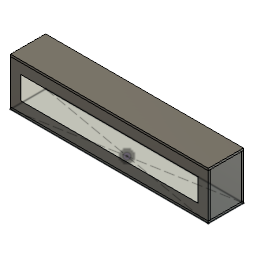
initial_3d_design (Autodesk Fusion 360 design; units mm, degrees)
part number: 2026-03-02-16-33-59-014
part number: 2026-03-03-11-30-51-863
part number: 2026-03-03-11-31-05-266
part number: 2026-03-03-11-31-17-109
part number: 2026-03-03-11-31-19-151
part number: 2026-03-03-11-31-20-913
part number: 2026-03-03-11-31-23-209
part number: 2026-03-03-11-31-25-857
part number: 2026-03-03-11-31-27-912
part number: 2026-03-03-11-31-30-099
Autodesk Fusion 360 part; units mm, degrees
sketch "Base/Top" plane through (0, 0, 0) normal (0, 1, 0) x (1, 0, 0)
  line L0 (143, 25.5) -> (-143, 25.5)
  line L1 (-143, 25.5) -> (-143, -25.5)
  line L2 (-143, -25.5) -> (143, -25.5)
  line L3 (143, -25.5) -> (143, 25.5)
  line L4 (143, 25.5) -> (-143, -25.5) construction
  line L5 (-143, 25.5) -> (143, -25.5) construction
  dimension "d12" = 286
  dimension "d13" = 51
  constraint horizontal L0
  constraint perpendicular L0 L1
  constraint parallel L0 L2
  constraint parallel L1 L3
  constraint coincident L4 origin
  constraint coincident L5 origin
  measures "d12" distance of L1.end L2.end
  measures "d13" distance of L0.end L1.end
sketch "Front" plane through (0, 0, 0) normal (0, 0, 1) x (1, 0, 0)
  line L0 (128, 16.5) -> (-128, 16.5)
  line L1 (-128, 16.5) -> (-128, -16.5)
  line L2 (-128, -16.5) -> (128, -16.5)
  line L3 (128, -16.5) -> (128, 16.5)
  line L4 (128, 16.5) -> (-128, -16.5) construction
  line L5 (-128, 16.5) -> (128, -16.5) construction
  line L6 (143, 31.5) -> (-143, 31.5)
  line L7 (-143, 31.5) -> (-143, -31.5)
  line L8 (-143, -31.5) -> (143, -31.5)
  line L9 (143, -31.5) -> (143, 31.5)
  line L10 (143, 31.5) -> (-143, -31.5) construction
  line L11 (-143, 31.5) -> (143, -31.5) construction
  dimension "d15" = 256
  dimension "d16" = 33
  dimension "d17" = 286
  dimension "d18" = 63
  constraint horizontal L0
  constraint perpendicular L0 L1
  constraint parallel L0 L2
  constraint parallel L1 L3
  constraint coincident L4 origin
  constraint coincident L5 origin
  constraint horizontal L6
  constraint perpendicular L6 L7
  constraint parallel L6 L8
  constraint parallel L7 L9
  constraint coincident L10 origin
  constraint coincident L11 origin
  measures "d15" distance of L1.end L2.end
  measures "d16" distance of L0.end L1.end
  measures "d17" distance of L7.end L8.end
  measures "d18" distance of L6.end L7.end
sketch "Lights" plane through (0, 0, 0) normal (0, 0, 1) x (1, 0, 0)
  line L0 (128, 16.5) -> (-128, 16.5)
  line L1 (-128, 16.5) -> (-128, -16.5)
  line L2 (-128, -16.5) -> (128, -16.5)
  line L3 (128, -16.5) -> (128, 16.5)
  line L4 (128, 16.5) -> (-128, -16.5) construction
  line L5 (-128, 16.5) -> (128, -16.5) construction
  line L6 (0, 0) -> (128, 0) construction
  line L7 (0, 0) -> (0, 16.5) construction
  dimension "d19" = 256
  dimension "d20" = 33
  constraint horizontal L0
  constraint perpendicular L0 L1
  constraint parallel L0 L2
  constraint parallel L1 L3
  constraint coincident L4 L6.start
  constraint coincident L5 L6.start
  constraint coincident L6.start L7.start
  constraint midpoint L3 L6.end
  constraint midpoint L0 L7.end
  measures "d19" distance of L1.end L2.end
  measures "d20" distance of L0.end L1.end
sketch "Back" plane through (0, 0, 0) normal (0, 0, 1) x (1, 0, 0)
  line L0 (143, 31.5) -> (-143, 31.5)
  line L1 (-143, 31.5) -> (-143, -31.5)
  line L2 (-143, -31.5) -> (143, -31.5)
  line L3 (143, -31.5) -> (143, 31.5)
  line L4 (143, 31.5) -> (-143, -31.5) construction
  line L5 (-143, 31.5) -> (143, -31.5) construction
  line L6 (143, -31.5) -> (128, -31.5) construction
  line L7 (128, -31.5) -> (128, -24) construction
  line L8 (128, -24) -> (118, -24)
  line L9 (118, -24) -> (118, -21.5)
  line L10 (118, -21.5) -> (128, -21.5)
  line L11 (128, -21.5) -> (128, -24)
  line L12 (118, -24) -> (110.5, -24) construction
  line L13 (110.5, -24) -> (98.5, -24)
  line L14 (98.5, -24) -> (98.5, -12)
  line L15 (98.5, -12) -> (110.5, -12)
  line L16 (110.5, -12) -> (110.5, -24)
  line L17 (128, -21.5) -> (123, -21.5) construction
  line L18 (123, -21.5) -> (123, -16.5) construction
  circle A0 centre (123, -16.5) radius 2.5
  dimension "d21" = 286
  dimension "d22" = 63
  dimension "d23" = 15
  dimension "d24" = 7.5
  dimension "d27" = 10
  dimension "d28" = 2.5
  dimension "d29" = 7.5
  dimension "d30" = 12
  dimension "d31" = 12
  dimension "d32" = 5
  dimension "d34" = 5
  constraint horizontal L0
  constraint perpendicular L0 L1
  constraint parallel L0 L2
  constraint parallel L1 L3
  constraint coincident L4 origin
  constraint coincident L5 origin
  constraint perpendicular L3 L6
  constraint perpendicular L2 L7
  constraint horizontal L8
  constraint vertical L9
  constraint horizontal L10
  constraint vertical L11
  constraint perpendicular L9 L12
  constraint horizontal L13
  constraint vertical L14
  constraint horizontal L15
  constraint vertical L16
  constraint midpoint L10 L17.end
  constraint perpendicular L17 L18
  constraint coincident L18.end A0.centre
  measures "d21" distance of L1.end L2.end
  measures "d22" distance of L0.end L1.end
  measures "d23" distance of L2.end L6.end
  measures "d24" distance of L6.end L7.end
  measures "d27" distance of L7.end L8.end
  measures "d28" distance of L7.end L10.end
  measures "d29" distance of L8.end L12.end
  measures "d30" distance of L12.end L13.end
  measures "d31" distance of L12.end L15.end
  measures "d32" distance of L17.end L18.end
  measures "d34" diameter of A0
sketch "Sides" plane through (0, 0, 0) normal (1, 0, 0) x (0, 0, -1)
  line L0 (22.5, 31.5) -> (-22.5, 31.5)
  line L1 (-22.5, 31.5) -> (-22.5, -31.5)
  line L2 (-22.5, -31.5) -> (22.5, -31.5)
  line L3 (22.5, -31.5) -> (22.5, 31.5)
  line L4 (22.5, 31.5) -> (-22.5, -31.5) construction
  line L5 (-22.5, 31.5) -> (22.5, -31.5) construction
  dimension "d35" = 45
  dimension "d36" = 63
  constraint horizontal L0
  constraint perpendicular L0 L1
  constraint parallel L0 L2
  constraint parallel L1 L3
  constraint coincident L4 origin
  constraint coincident L5 origin
  measures "d35" distance of L1.end L2.end
  measures "d36" distance of L0.end L1.end
sketch "Esp32" plane through (0, 0, 0) normal (0, 1, 0) x (1, 0, 0)
  line L0 (-28.5, -14.25) -> (28.5, -14.25)
  line L1 (28.5, -14.25) -> (28.5, 14.25)
  line L2 (28.5, 14.25) -> (-28.5, 14.25)
  line L3 (-28.5, 14.25) -> (-28.5, -14.25)
  line L4 (-28.5, -14.25) -> (28.5, 14.25) construction
  line L5 (28.5, -14.25) -> (-28.5, 14.25) construction
  dimension "d37" = 57
  dimension "d38" = 28.5
  constraint horizontal L0
  constraint perpendicular L0 L1
  constraint parallel L0 L2
  constraint parallel L1 L3
  constraint coincident L4 origin
  constraint coincident L5 origin
  measures "d37" distance of L1.end L2.end
  measures "d38" distance of L0.end L1.end
sketch "Button" plane through (0, 0, 0) normal (0, 0, 1) x (1, 0, 0)
  line L0 (-6, 6) -> (6, 6)
  line L1 (6, 6) -> (6, -6)
  line L2 (6, -6) -> (-6, -6)
  line L3 (-6, -6) -> (-6, 6)
  line L4 (-6, 6) -> (6, -6) construction
  line L5 (6, 6) -> (-6, -6) construction
  circle A0 centre (0, 0) radius 2.6
  dimension "d39" = 12
  dimension "d40" = 12
  dimension "d41" = 5.2
  constraint horizontal L0
  constraint perpendicular L0 L1
  constraint parallel L0 L2
  constraint parallel L1 L3
  constraint coincident L4 A0.centre
  constraint coincident L5 A0.centre
  constraint coincident A0.centre origin
  measures "d39" distance of L1.end L2.end
  measures "d40" distance of L0.end L1.end
  measures "d41" diameter of A0
extrude "Extrude1" add sketch "Base/Top" along normal blind 3 makes body 1
copy_body "CopyPasteBodies1" bodies 1 makes body 2
extrude "Extrude2" add sketch "Front" along normal blind 3 separate body makes body 3
extrude "Extrude3" add sketch "Lights" along normal blind 15 separate body makes body 4
extrude "Extrude4" add sketch "Back" along normal blind 3 separate body makes body 5
extrude "Extrude5" add sketch "Sides" along normal blind 3 separate body makes body 6
copy_body "CopyPasteBodies2" bodies 6 makes body 7
extrude "Extrude6" add sketch "Esp32" along normal blind 3 separate body makes body 8
extrude "Extrude7" add sketch "Button" along normal blind 6.5 separate body makes body 9
extrude "Extrude8" add sketch "Button" along normal blind 8.5 separate body contours A0 makes body 10
combine "Combine1" operation add target body 9 tool bodies 10
copy_body "Body->Comp1" bodies 1 removing the originals makes body 11 in component "Base"
copy_body "Body->Comp2" bodies 3 removing the originals makes body 12 in component "Front"
copy_body "Body->Comp3" bodies 2 removing the originals makes body 13 in component "Top"
copy_body "Body->Comp4" bodies 4 removing the originals makes body 14 in component "Lights"
copy_body "Body->Comp5" bodies 5 removing the originals makes body 15 in component "Back"
copy_body "Body->Comp6" bodies 6 removing the originals makes body 16 in component "LeftSide"
copy_body "Body->Comp7" bodies 7 removing the originals makes body 17 in component "RightSide"
copy_body "Body->Comp8" bodies 8 removing the originals makes body 18 in component "ESP32"
copy_body "Body->Comp9" bodies 9 removing the originals makes body 19 in component "Button"
fillet "Fillet1" radius 1 4 edges at (118, -21.5, 1.5) (118, -24, 1.5) (128, -24, 1.5) (128, -21.5, 1.5) on bodies 15 in component "Back"
fillet "Fillet1'" radius 1 4 edges at (0, -6, 6.5) (6, 0, 6.5) (-6, 0, 6.5) (0, 6, 6.5) on bodies 19 in component "Button"
move_body "Move1" bodies 18 to x (1, 0, 0) y (0, 1, 0) z (0, 0, 1) at (0, 100, 0) in component "ESP32"
move_body "Move1'" bodies 13 to x (1, 0, 0) y (0, 1, 0) z (0, 0, 1) at (0, 90, 0) in component "Top"
component "Base" placed x (1, 0, 0) y (0, 1, 0) z (0, 0, 1) at (0, 0, 0)
component "Front" placed x (1, 0, 0) y (0, 1, 0) z (0, 0, 1) at (0, 34.5, 22.5)
component "Top" placed x (1, 0, 0) y (0, 1, 0) z (0, 0, 1) at (0, -24, 0)
component "Lights" placed x (1, 0, 0) y (0, 1, 0) z (0, 0, 1) at (0, 34.5, 10.5)
component "Back" placed x (-1, 0, 0) y (0, 1, 0) z (0, 0, -1) at (0, 34.5, -22.5)
component "LeftSide" placed x (1, 0, 0) y (0, 1, 0) z (0, 0, 1) at (-143, 34.5, 0)
component "RightSide" placed x (1, 0, 0) y (0, 1, 0) z (0, 0, 1) at (140, 34.5, 0)
component "ESP32" placed x (1, 0, 0) y (0, 1, 0) z (0, 0, 1) at (-111.5, -97, -4.25)
component "Button" placed x (-1, 0, 0) y (0, 1, 0) z (0, 0, -1) at (-104.5, 16.5, -20)
equation "lights_length = 256 mm"
equation "lights_width = 33 mm"
equation "lights_depth = 15 mm"
equation "housing_buffer = 15 mm"
equation "mat_thickness = 3 mm"
equation "esp32_length = 57 mm"
equation "esp32_width = 28.5 mm"
equation "button_base_w = 12 mm"
equation "button_d = 5.2 mm"
equation "button_base_depth = 6.5 mm"
equation "button_height = 2 mm"
equation "d12 = lights_length + housing_buffer * 2"
equation "d13 = lights_depth + 2 * housing_buffer + 2 * mat_thickness"
equation "d15 = lights_length"
equation "d16 = lights_width"
equation "d17 = lights_length + ( 2 * housing_buffer )"
equation "d18 = lights_width + ( housing_buffer * 2 )"
equation "d19 = lights_length"
equation "d20 = lights_width"
equation "d21 = lights_length + ( 2 * housing_buffer )"
equation "d22 = lights_width + ( 2 * housing_buffer )"
equation "d23 = housing_buffer"
equation "d24 = housing_buffer / 2"
equation "usb_length = 10 mm"
equation "usb_height = 2.5 mm"
equation "d27 = usb_length"
equation "d28 = usb_height"
equation "d29 = housing_buffer / 2"
equation "d30 = button_base_w"
equation "d31 = button_base_w"
equation "d32 = usb_height + led_d / 2"
equation "led_d = 5 mm"
equation "d34 = led_d"
equation "d35 = lights_depth + ( 2 * housing_buffer )"
equation "d36 = lights_width + ( 2 * housing_buffer )"
equation "d37 = esp32_length"
equation "d38 = esp32_width"
equation "d39 = button_base_w"
equation "d40 = button_base_w"
equation "d41 = button_d"
equation "d42 = mat_thickness"
equation "d44 = mat_thickness"
equation "d46 = lights_depth"
equation "d48 = mat_thickness"
equation "d50 = mat_thickness"
equation "d52 = mat_thickness"
equation "d54 = button_base_depth"
equation "d56 = button_base_depth + button_height"
named bodies: "Base", "Top", "Front", "Lights", "Back", "LeftSide", "RightSide", "ESP32", "Button"
